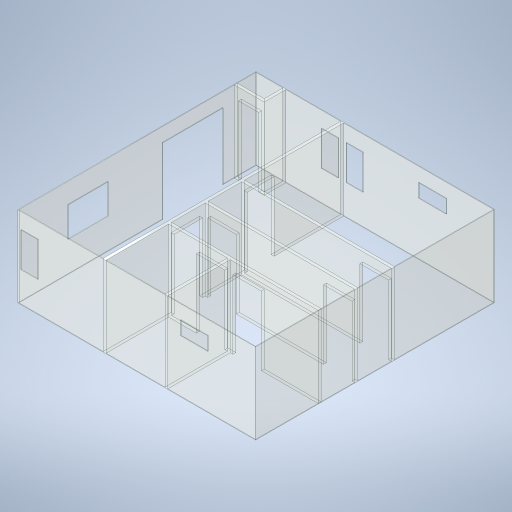
# Autodesk Inventor part: Interior_Walls
Saved by Autodesk Inventor 2024.1 (Build 281209000, 209)
## iProperties
Created: 2023-05-16
Part Number: Interior_Walls
Material: Wood (Southern Pine)
Document SubType Name: Modeling
Designer: Tom
Density: 0.420735 g/cm^3
Appearance: Clear
Mass: 7.46669e+07 g
Surface Area: 2.27384e+06 cm^2
Volume: 9.51171e+06 cm^3
Author: Tom
Autodesk Inventor part; units mm, degrees
ref_plane "YZ Plane" through (0, 0, 0) normal (1, 0, 0) x (0, 1, 0)
ref_plane "XZ Plane" through (0, 0, 0) normal (0, 1, 0) x (-1, 0, 0)
ref_plane "XY Plane" through (0, 0, 0) normal (0, 0, 1) x (1, 0, 0)
sketch "Sketch1" plane through (0, 0, 0) normal (0, 1, 0) x (-1, 0, 0)
  line L0 (3606.8, -3606.8) -> (-3606.8, -3606.8)
  line L1 (-3606.8, -3606.8) -> (-3594.1, 3606.8)
  line L2 (-3594.1, 3606.8) -> (3594.1, 3606.8)
  line L3 (3594.1, 3606.8) -> (3606.8, -3606.8)
  line L4 (0, -3606.8) -> (0, 3606.8)
  line L5 (3600.45, 0) -> (-3600.45, 0)
  line L6 (3575.0835, 3587.75) -> (-3575.0835, 3587.75)
  line L7 (-3575.0835, 3587.75) -> (-3587.7164, -3587.75)
  line L8 (-3587.7164, -3587.75) -> (3587.7164, -3587.75)
  line L9 (3587.7164, -3587.75) -> (3575.0835, 3587.75)
  line L10 (-2204.4316, 514.35) -> (-2204.4316, 603.25)
  line L11 (5.3684, -603.25) -> (5.3684, -514.35)
  point P0 (0, 0)
  point P1 (0, 0)
  point P2 (-3581.4, 0)
  dimension "d1" = 7213.6
  dimension "d2" = 12.7
  dimension "d4" = 7188.2
  dimension "d5" = 7213.6
  dimension "d6" = 19.05
  constraints: 24 end point, 6 midpoint, 2 parallel, 1 coincident, 1 horizontal, 1 perpendicular, 3 other
  measures "d1" distance of L0.start L0.end
  measures "d2" horizontal distance of L0.start L2.end
  measures "d4" distance of L1.end L2.end
  measures "d5" distance of L0.end L1.end
  measures "d6" distance between parallel lines of L2 L6
extrude "Extrusion1" add sketch "Sketch1" along normal blind 2438.4 contours L0 L4 L8 L9 L5 L3 | L0 L1 L5 L7 L8 L4 | L5 L9 L6 L4 L2 L3 | L1 L2 L4 L6 L7 L5
sketch "Sketch2" plane through (0, 2438.4, 0) normal (0, 1, 0) x (1, 0, 0)
  line L0 (-3587.7164, 3587.75) -> (3587.7164, 3587.75) projected
  line L1 (3575.0835, -3587.75) -> (-3575.0835, -3587.75) projected
  line L2 (-3587.7164, 3587.75) -> (3587.7164, 3587.75) projected
  line L3 (3575.0835, -3587.75) -> (-3575.0835, -3587.75) projected
  line L4 (3587.7164, 3587.75) -> (3575.0835, -3587.75) projected
  line L5 (-939.7665, -1612.9) -> (3578.4038, -1612.9)
  line L6 (3578.4038, -1612.9) -> (3578.4038, -1701.8)
  line L7 (3578.4038, -1701.8) -> (-939.7665, -1701.8)
  line L8 (927.1335, -1701.8) -> (838.2335, -1701.8)
  line L9 (838.2335, -1701.8) -> (838.2335, -3587.75)
  line L10 (838.2335, -3587.75) -> (927.1335, -3587.75)
  line L11 (927.1335, -3587.75) -> (927.1335, -1701.8)
  line L12 (-939.7665, -3587.75) -> (-939.7665, 3587.75)
  line L13 (-1028.6665, 3587.75) -> (-1028.6665, -3587.75)
  line L14 (-939.7665, 3587.75) -> (-1028.6665, 3587.75)
  line L15 (-939.7665, -3587.75) -> (-1028.6665, -3587.75)
  line L16 (-939.7665, -533.4) -> (-939.7665, -444.5)
  line L17 (-3575.0835, -3587.75) -> (-3587.7164, 3587.75) projected
  line L18 (-3586.5649, 2933.7) -> (-2684.8649, 2933.7)
  line L19 (-2773.7649, 3022.6) -> (-3586.5649, 3022.6)
  line L20 (-3586.5649, 3022.6) -> (-3586.5649, 2933.7)
  line L21 (-2773.7649, 3022.6) -> (-2773.7649, 3587.75)
  line L22 (-2773.7649, 3587.75) -> (-2684.8649, 3587.75)
  line L23 (-2684.8649, 3587.75) -> (-2684.8649, 2933.7)
  line L24 (-939.7665, -596.9) -> (3580.5056, -596.9)
  line L25 (3580.5056, -596.9) -> (3580.5056, -508)
  line L26 (3580.5056, -508) -> (-939.7665, -508)
  line L27 (-939.7665, -508) -> (-939.7665, -596.9)
  line L28 (-939.7665, -1701.8) -> (-939.7665, -1612.9)
  line L29 (-939.7665, 508) -> (3582.4509, 508)
  line L30 (3582.4509, 508) -> (3582.4509, 596.9)
  line L31 (3582.4509, 596.9) -> (-939.7665, 596.9)
  line L32 (-939.7665, 596.9) -> (-939.7665, 508)
  point P0 (0, 0)
  point P1 (838.2335, -1701.8)
  point P2 (-1028.6665, -3587.75)
  point P3 (-939.7665, 3587.75)
  point P4 (-2684.8649, 3587.75)
  point P5 (-2773.7649, 3587.75)
  point P6 (-939.7665, 596.9)
  point P7 (-939.7665, -508)
  dimension "d41" = 88.9
  dimension "d44" = 2647.95
  dimension "d45" = 1778
  dimension "d90" = 812.8
  dimension "d137" = 1016
  dimension "d138" = 508
  dimension "d139" = 508
  dimension "d185" = 654.05
  constraints: 54 end point, 16 point on line, 10 parallel, 9 perpendicular, 7 equal length, 5 horizontal, 2 collinear
  measures "d41" distance between parallel lines of L13 L12
  measures "d44" distance from line of L1.start L11
  measures "d45" distance between parallel lines of L9 L12
  measures "d90" distance of L19.start L19.end
  measures "d137" distance between parallel lines of L5 L24
  measures "d138" distance from line of point (0, 0) L26
  measures "d139" distance from line of L29 point (0, 0)
  measures "d185" distance of L22.end L18.end
extrude "Extrusion2" add sketch "Sketch2" against normal blind 2438.4 contours L0 L23 L18 L20 L19 L21 | L0 L12 L1 L13 | L31 L4 L29 L12 | L9 L7 L11 L1 | L12 L5 L6 L7 | L30 L29 L4 | L12 L26 L4 L24 | L25 L24 L4
sketch "Sketch5" plane through (-3594.1, 0, 3606.8) normal (0, 0, 1) x (1, 0, 0)
  line L0 (4914.9, 2006.6) -> (5740.4, 2006.6)
  line L1 (5740.4, 2006.6) -> (5740.4, 1600.2)
  line L2 (5740.4, 1600.2) -> (4914.9, 1600.2)
  line L3 (4914.9, 1600.2) -> (4914.9, 2006.6)
  line L4 (0, 0) -> (7188.2, 0) projected
  line L5 (7188.2, 0) -> (7188.2, 2438.4) projected
  point P0 (3594.1, 0)
  dimension "d51" = 2006.6
  dimension "d53" = 825.5
  dimension "d54" = 406.4
  dimension "d166" = 1447.8
  constraints: 8 end point, 2 parallel, 1 horizontal, 1 perpendicular
  measures "d51" distance between parallel lines of L4 L0
  measures "d53" distance of L0.start L0.end
  measures "d54" distance between parallel lines of L2 L0
  measures "d166" distance between parallel lines of L5 L1
extrude "Extrusion4" cut sketch "Sketch5" against normal up to surface (19.05 mm away)
sketch "Sketch6" plane through (3606.8, 0, -3606.8) normal (0, 0, -1) x (-1, 0, 0)
  line L0 (1447.8, 2006.6) -> (2286, 2006.6)
  line L1 (2286, 2006.6) -> (2286, 1600.2)
  line L2 (2286, 1600.2) -> (1447.8, 1600.2)
  line L3 (1447.8, 1600.2) -> (1447.8, 2006.6)
  line L4 (0, 0) -> (7213.6, 0) projected
  line L5 (0, 0) -> (0, 2438.4) projected
  point P0 (3606.8, 0)
  point P1 (1447.8, 1803.4)
  dimension "d57" = 2006.6
  dimension "d58" = 406.4
  dimension "d59" = 838.2
  dimension "d60" = 1447.8
  constraints: 8 end point, 2 parallel, 1 horizontal, 1 midpoint, 1 perpendicular
  measures "d57" distance between parallel lines of L4 L0
  measures "d58" distance of L2.end L0.start
  measures "d59" distance of L1.end L2.end
  measures "d60" distance from line of L5 point (1447.8, 1803.4)
extrude "Extrusion5" cut sketch "Sketch6" against normal up to surface (19.05 mm away)
sketch "Sketch7" plane through (-3587.7164, 0, -3587.75) normal (0.9999985, 0, -0.0017606) x (-0.0017606, 0, -0.9999985)
  line L0 (-996.95, 0) -> (-2825.75, 0)
  line L1 (-2825.75, 0) -> (-2825.75, 2006.6)
  line L2 (-2825.75, 2006.6) -> (-996.95, 2006.6)
  line L3 (-996.95, 2006.6) -> (-996.95, 0)
  line L4 (0, 0) -> (0, 2438.4) projected
  line L5 (-7175.5111, 0) -> (-654.051, 0) projected
  point P0 (-3594.0608, 0)
  dimension "d63" = 996.95
  dimension "d64" = 2006.6
  dimension "d65" = 1828.8
  constraints: 8 end point, 2 parallel, 1 collinear, 1 horizontal, 1 perpendicular
  measures "d63" distance between parallel lines of L3 L4
  measures "d64" distance of L0.end L1.end
  measures "d65" distance of L1.end L2.end
extrude "Extrusion6" cut sketch "Sketch7" against normal up to surface (19.05 mm away)
sketch "Sketch8" plane through (-3594.1, 0, 3606.8) normal (-0.9999985, 0, 0.0017606) x (0.0017606, 0, 0.9999985)
  line L0 (-2717.8, 1816.1) -> (-1511.3, 1816.1)
  line L1 (-1511.3, 1816.1) -> (-1511.3, 914.4)
  line L2 (-1511.3, 914.4) -> (-2717.8, 914.4)
  line L3 (-2717.8, 914.4) -> (-2717.8, 1816.1)
  line L4 (0, 0) -> (0, 2438.4) projected
  line L5 (-7213.6112, 0) -> (0, 0) projected
  point P0 (-3600.4668, 0)
  point P1 (-4368.7776, 0)
  dimension "d71" = 2717.8
  dimension "d72" = 901.7
  dimension "d73" = 1206.5
  dimension "d111" = 914.4
  constraints: 8 end point, 2 parallel, 1 horizontal, 1 perpendicular
  measures "d71" distance between parallel lines of L3 L4
  measures "d72" distance of L0.end L1.end
  measures "d73" distance of L1.end L2.end
  measures "d111" distance from line of L5 L2.end
extrude "Extrusion7" cut sketch "Sketch8" against normal up to surface (19.05 mm away)
sketch "Sketch9" plane through (3587.7164, 0, -3587.75) normal (0, 0, 1) x (1, 0, 0)
  line L0 (-4451.2829, 1955.8) -> (-3943.2829, 1955.8)
  line L1 (-3943.2829, 1955.8) -> (-3943.2829, 914.4)
  line L2 (-3943.2829, 914.4) -> (-4451.2829, 914.4)
  line L3 (-4451.2829, 914.4) -> (-4451.2829, 1955.8)
  line L4 (-7175.4329, 0) -> (0, 0) projected
  line L5 (-4527.4829, 2438.4) -> (-4527.4829, 0) projected
  point P0 (-3587.7164, 0)
  dimension "d76" = 1041.4
  dimension "d77" = 914.4
  dimension "d78" = 76.2
  dimension "d79" = 508
  constraints: 8 end point, 2 parallel, 1 horizontal, 1 perpendicular
  measures "d76" distance of L0.end L1.end
  measures "d77" distance between parallel lines of L4 L2
  measures "d78" distance between parallel lines of L5 L3
  measures "d79" distance of L0.start L0.end
extrude "Extrusion8" cut sketch "Sketch9" against normal up to surface (19.05 mm away)
sketch "Sketch10" plane through (-3587.7164, 0, -3587.75) normal (0, 0, 1) x (1, 0, 0)
  line L0 (2482.8499, 914.4) -> (1974.8499, 914.4)
  line L1 (1974.8499, 914.4) -> (1974.8499, 1955.8)
  line L2 (1974.8499, 1955.8) -> (2482.8499, 1955.8)
  line L3 (2482.8499, 1955.8) -> (2482.8499, 914.4)
  line L4 (2559.0499, 0) -> (2559.0499, 2438.4) projected
  line L5 (0, 0) -> (7175.4329, 0) projected
  point P0 (3587.7164, 0)
  dimension "d82" = 76.2
  dimension "d83" = 914.4
  dimension "d84" = 508
  dimension "d85" = 1041.4
  constraints: 8 end point, 2 parallel, 1 horizontal, 1 perpendicular
  measures "d82" distance between parallel lines of L4 L3
  measures "d83" distance between parallel lines of L5 L0
  measures "d84" distance of L1.end L2.end
  measures "d85" distance of L0.end L1.end
extrude "Extrusion9" cut sketch "Sketch10" against normal up to surface (19.05 mm away)
sketch "Sketch11" plane through (-3586.5649, 2438.4, -2933.7) normal (0, 0, 1) x (1, 0, 0)
  line L0 (0, -2438.4) -> (812.8, -2438.4) projected
  line L1 (736.6, -2438.4) -> (127, -2438.4)
  line L2 (127, -2438.4) -> (127, -355.6)
  line L3 (127, -355.6) -> (736.6, -355.6)
  line L4 (736.6, -355.6) -> (736.6, -2438.4)
  line L5 (901.7, 0) -> (901.7, -2438.4) projected
  point P0 (3586.5649, -2438.4)
  dimension "d91" = 165.1
  dimension "d92" = 609.6
  dimension "d95" = 2082.8
  constraints: 8 end point, 2 parallel, 1 horizontal, 1 perpendicular, 1 point on line
  measures "d91" distance between parallel lines of L5 L4
  measures "d92" distance of L2.end L3.end
  measures "d95" distance of L1.end L2.end
extrude "Extrusion10" cut sketch "Sketch11" against normal up to surface (88.9 mm away)
sketch "Sketch12" plane through (-939.7665, 2438.4, 1701.8) normal (0, 0, 1) x (1, 0, 0)
  line L0 (1778, -2438.4) -> (0, -2438.4) projected
  line L1 (1701.8, -2438.4) -> (838.2, -2438.4)
  line L2 (838.2, -2438.4) -> (838.2, -355.6)
  line L3 (838.2, -355.6) -> (1701.8, -355.6)
  line L4 (1701.8, -355.6) -> (1701.8, -2438.4)
  line L5 (1778, 0) -> (1778, -2438.4) projected
  point P0 (939.7665, -2438.4)
  dimension "d96" = 76.2
  dimension "d97" = 863.6
  dimension "d98" = 2082.8
  constraints: 8 end point, 2 parallel, 1 horizontal, 1 perpendicular, 1 point on line
  measures "d96" distance between parallel lines of L5 L4
  measures "d97" distance of L2.end L3.end
  measures "d98" distance of L1.end L2.end
extrude "Extrusion11" cut sketch "Sketch12" against normal up to surface (88.9 mm away)
sketch "Sketch15" plane through (-3594.1, 0, 3606.8) normal (0, 0, 1) x (1, 0, 0)
  line L0 (95.2165, 1955.8) -> (603.2165, 1955.8)
  line L1 (603.2165, 1955.8) -> (603.2165, 914.4)
  line L2 (603.2165, 914.4) -> (95.2165, 914.4)
  line L3 (95.2165, 914.4) -> (95.2165, 1955.8)
  line L4 (0, 0) -> (7188.2, 0) projected
  point P0 (3594.1, 0)
  point P1 (19.0165, 2438.4)
  dimension "d113" = 1041.4
  dimension "d114" = 508
  dimension "d115" = 76.2
  dimension "d116" = 914.4
  constraints: 8 end point, 2 parallel, 1 horizontal, 1 perpendicular
  measures "d113" distance of L0.end L1.end
  measures "d114" distance of L0.start L0.end
  measures "d115" distance from line of L3 point (19.016, 2438.4)
  measures "d116" distance between parallel lines of L4 L2
extrude "Extrusion14" cut sketch "Sketch15" against normal up to surface (19.05 mm away)
sketch "Sketch16" plane through (-1028.6665, 2438.4, -3587.75) normal (-1, 0, 0) x (0, 0, 1)
  line L0 (5200.65, 0) -> (5200.65, -2438.4) projected
  line L1 (4121.15, 0) -> (4121.15, -2438.4) projected
  line L2 (7175.5, -2438.4) -> (0, -2438.4) projected
  line L3 (5124.45, -2438.4) -> (4260.85, -2438.4)
  line L4 (4260.85, -2438.4) -> (4260.85, -355.6)
  line L5 (4260.85, -355.6) -> (5124.45, -355.6)
  line L6 (5124.45, -355.6) -> (5124.45, -2438.4)
  point P0 (3587.75, -2438.4)
  point P1 (7035.8, -2470.15)
  point P2 (0, -2470.15)
  point P3 (0, -2438.4)
  dimension "d122" = 76.2
  dimension "d123" = 863.6
  dimension "d124" = 2082.8
  constraints: 8 end point, 2 parallel, 1 horizontal, 1 perpendicular, 2 other
  measures "d122" distance between parallel lines of L0 L6
  measures "d123" distance of L4.end L5.end
  measures "d124" distance of L3.end L4.end
extrude "Extrusion15" cut sketch "Sketch16" against normal up to surface (88.9 mm away)
sketch "Sketch22" plane through (-939.7665, 2438.4, -596.9) normal (1, 0, 0) x (0, 0, -1)
  line L0 (2990.85, -2438.4) -> (0, -2438.4) projected
  line L1 (76.2, -2438.4) -> (889, -2438.4)
  line L2 (889, -2438.4) -> (889, -355.6)
  line L3 (889, -355.6) -> (76.2, -355.6)
  line L4 (76.2, -355.6) -> (76.2, -2438.4)
  line L5 (0, 0) -> (0, -2438.4) projected
  point P0 (-596.9, -2438.4)
  dimension "d156" = 812.8
  dimension "d157" = 2082.8
  dimension "d184" = 76.2
  constraints: 8 end point, 2 parallel, 1 horizontal, 1 perpendicular, 1 point on line
  measures "d156" distance of L2.end L3.end
  measures "d157" distance of L1.end L2.end
  measures "d184" distance between parallel lines of L5 L4
extrude "Extrusion21" cut sketch "Sketch22" against normal up to surface (88.9 mm away)
sketch "Sketch23" plane through (-939.7665, 2438.4, 596.9) normal (0, 0, 1) x (1, 0, 0)
  line L0 (76.2, -2438.4) -> (939.8, -2438.4)
  line L1 (939.8, -2438.4) -> (939.8, -355.6)
  line L2 (939.8, -355.6) -> (76.2, -355.6)
  line L3 (76.2, -355.6) -> (76.2, -2438.4)
  line L4 (4520.1156, -2438.4) -> (0, -2438.4) projected
  point P0 (939.7665, -2438.4)
  point P1 (0, 0)
  dimension "d160" = 76.2
  dimension "d161" = 2082.8
  dimension "d162" = 863.6
  constraints: 8 end point, 2 parallel, 1 collinear, 1 horizontal, 1 perpendicular
  measures "d160" distance from line of point (0, 0) L3
  measures "d161" distance of L0.end L1.end
  measures "d162" distance of L1.end L2.end
extrude "Extrusion22" cut sketch "Sketch23" against normal up to surface (88.9 mm away)
sketch "Sketch24" plane through (927.1335, 2438.4, 1701.8) normal (0, 0, 1) x (1, 0, 0)
  line L0 (2651.2703, -2438.4) -> (0, -2438.4) projected
  line L1 (76.2, -2438.4) -> (939.8, -2438.4)
  line L2 (939.8, -2438.4) -> (939.8, -355.6)
  line L3 (939.8, -355.6) -> (76.2, -355.6)
  line L4 (76.2, -355.6) -> (76.2, -2438.4)
  line L5 (0, -2438.4) -> (0, 0) projected
  point P0 (-927.1335, -2438.4)
  point P1 (939.8, -2438.4)
  dimension "d169" = 76.2
  dimension "d170" = 863.6
  dimension "d171" = 2082.8
  constraints: 8 end point, 2 parallel, 1 horizontal, 1 perpendicular, 1 point on line
  measures "d169" distance between parallel lines of L5 L4
  measures "d170" distance between parallel lines of L2 L4
  measures "d171" distance of L1.end L2.end
extrude "Extrusion24" cut sketch "Sketch24" against normal up to surface (88.9 mm away)
sketch "Sketch25" plane through (-939.7665, 2438.4, 596.9) normal (0, 0, 1) x (1, 0, 0)
  line L0 (4546.5665, -2438.4) -> (-2667.0335, -2438.4) projected
  line L1 (3575.05, -2438.4) -> (4438.65, -2438.4)
  line L2 (4438.65, -2438.4) -> (4438.65, -355.6)
  line L3 (4438.65, -355.6) -> (3575.05, -355.6)
  line L4 (3575.05, -355.6) -> (3575.05, -2438.4)
  line L5 (4514.85, -2438.4) -> (4514.85, 0) projected
  point P0 (939.7665, -2438.4)
  dimension "d174" = 76.2
  dimension "d175" = 2082.8
  dimension "d176" = 863.6
  constraints: 8 end point, 2 parallel, 1 horizontal, 1 perpendicular, 1 point on line
  measures "d174" distance between parallel lines of L5 L2
  measures "d175" distance of L1.end L2.end
  measures "d176" distance of L2.end L3.end
extrude "Extrusion25" cut sketch "Sketch25" against normal up to surface (88.9 mm away)
sketch "Sketch26" plane through (3582.4509, 2438.4, -596.9) normal (0, 0, -1) x (-1, 0, 0)
  line L0 (4522.2173, -2438.4) -> (0, -2438.4) projected
  line L1 (83.5673, -2438.4) -> (947.1673, -2438.4)
  line L2 (947.1673, -2438.4) -> (947.1673, -355.6)
  line L3 (947.1673, -355.6) -> (83.5673, -355.6)
  line L4 (83.5673, -355.6) -> (83.5673, -2438.4)
  line L5 (7.3673, -2438.4) -> (7.3673, 0) projected
  point P0 (3582.4509, -2438.4)
  point P1 (947.1673, -2438.4)
  dimension "d179" = 76.2
  dimension "d180" = 2082.8
  dimension "d181" = 863.6
  constraints: 8 end point, 2 parallel, 1 horizontal, 1 perpendicular, 1 point on line
  measures "d179" distance between parallel lines of L5 L4
  measures "d180" distance of L1.end L2.end
  measures "d181" distance of L2.end L3.end
extrude "Extrusion26" cut sketch "Sketch26" against normal up to surface (88.9 mm away)
body "Solid1"
